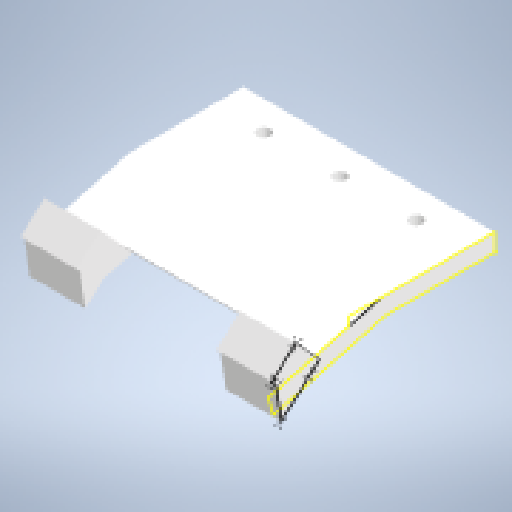
# Autodesk Inventor part: chest_cover_front
Saved by Autodesk Inventor 2026.1 (Build 301233020, 233B)
## iProperties
Created: 2026-01-21
Part Number: chest_cover_front
Material: 一般
Document SubType Name: Modeling
Designer: hibik
Density: 1 g/cm^3
Appearance: 既定
Author: hibik
Autodesk Inventor part; units mm, degrees
ref_plane "YZ Plane" through (0, 0, 0) normal (1, 0, 0) x (0, 1, 0)
ref_plane "XZ Plane" through (0, 0, 0) normal (0, 1, 0) x (-1, 0, 0)
ref_plane "XY Plane" through (0, 0, 0) normal (0, 0, 1) x (1, 0, 0)
sketch "スケッチ1" plane through (0, 0, 0) normal (0, 1, 0) x (-1, 0, 0)
  line L0 (21.5, 0) -> (-21.5, 0)
  line L1 (-21.5, 0) -> (-21.5, 25)
  line L2 (-21.5, 25) -> (21.5, 25)
  line L3 (21.5, 25) -> (21.5, 0)
  circle A0 centre (0, 5) radius 1.1
  circle A1 centre (13, 5) radius 1.1
  circle A2 centre (-13, 5) radius 1.1
  line L4 (0, 0) -> (0, 25) construction
  dimension "d0" = 43
  dimension "d1" = 13
  dimension "d2" = 2.2
  dimension "d3" = 5
  dimension "d6" = 25
  constraints: 10 end point, 3 centre point, 2 horizontal alignment, 2 midpoint, 2 parallel, 1 coincident, 1 equal radius, 1 horizontal, 1 perpendicular, 1 vertical alignment, 1 other
  measures "d0" distance of L1.end L2.end
  measures "d1" distance of A1.centre A0.centre
  measures "d2" diameter of A1
  measures "d3" distance from line of L0 A1.centre
  measures "d6" distance of L2.end L0.start
extrude "押し出し1" add sketch "スケッチ1" along normal blind 3
sketch "スケッチ2" plane through (21.5, 0, 25) normal (1, 0, 0) x (0, 0, -1)
  line L0 (5.6249, 3) -> (6.4287, 0)
  line L1 (6.4287, 0) -> (-12.8898, -5.1764)
  line L2 (-12.8898, -5.1764) -> (-13.6936, -2.1764)
  line L3 (-13.6936, -2.1764) -> (5.6249, 3)
  line L4 (0, 3) -> (25, 3) projected
  line L5 (0, 0) -> (25, 0) projected
  line L6 (6.134, 1.1) -> (-6.5703, -2.3041) construction
  dimension "d7" = 20
  constraints: 10 end point, 3 perpendicular, 3 point on line, 1 parallel, 2 other
  measures "d7" distance from line of L0.start L2
extrude "押し出し2" add sketch "スケッチ2" against normal up to surface (43 mm away)
sketch "スケッチ3" plane through (21.5, 0, 0) normal (1, 0, 0) x (0, 0, -1)
  line L0 (-36.517, -6.8159) -> (-30.0178, -0.888)
  line L1 (-30.0178, -0.888) -> (-34.0611, 3.545)
  line L2 (-34.0611, 3.545) -> (-38.1247, -0.1614)
  line L3 (-38.1247, -0.1614) -> (-37.4508, -0.9002)
  line L4 (-37.4508, -0.9002) -> (-36.517, -6.8159)
  line L5 (-25, 3) -> (0, 3) projected
  line L6 (-25, 1.4928) -> (-25, 3) projected
  line L7 (-25, 1.4928) -> (-38.6936, -2.1764) projected
  line L8 (-38.6936, -2.1764) -> (-37.8898, -5.1764) projected
  line L9 (-37.8898, -5.1764) -> (-18.5713, 0) projected
  line L10 (-18.5713, 0) -> (0, 0) projected
  line L11 (0, 0) -> (0, 3) projected
  line L12 (-25, 1.4928) -> (-19.3751, 3)
  line L13 (-25, 1.4928) -> (-38.6936, -2.1764) projected
  point P0 (0, 0)
  point P1 (-31.5703, -2.3041)
  point P2 (-36.821, -4.89)
  point P3 (-37.308, -1.8051)
  point P4 (-33.4007, -3.9735)
  point P5 (-30.7774, -0.0552)
  constraints: 12 end point, 3 perpendicular, 1 collinear, 1 point on line, 5 other
extrude "押し出し3" cut sketch "スケッチ3" against normal through all contours L9 L8 L7 L4 | L6 L5 L12
extrude "押し出し4" add sketch "スケッチ3" against normal up to surface (43 mm away) contours L4 L9 L0 | L4 L3 L2 L1 L7
sketch "スケッチ4" plane through (0, 0, 0) normal (1, 0, 0) x (0, 1, 0)
  line L0 (-0.9002, 37.4508) -> (-6.8159, 36.517) projected
  line L1 (-6.8159, 36.517) -> (-3.9735, 33.4007) projected
  line L2 (-3.9735, 33.4007) -> (0, 18.5713) projected
  line L3 (0, 18.5713) -> (0, 0) projected
  line L4 (0, 0) -> (3, 0) projected
  line L5 (3, 19.3751) -> (3, 0) projected
  line L6 (3, 19.3751) -> (-0.0552, 30.7774) projected
  line L7 (-0.0552, 30.7774) -> (3.545, 34.0611) projected
  line L8 (3.545, 34.0611) -> (-0.1614, 38.1247) projected
  line L9 (-0.1614, 38.1247) -> (-0.9002, 37.4508) projected
  line L10 (-0.0552, 30.7774) -> (-2.6391, 28.4206)
  point P0 (0, 0)
  constraints: 2 end point, 1 point on line
extrude "押し出し5" cut sketch "スケッチ4" along normal mid plane 24 contours L9 L8 L7 L10 L2 L1 L0
